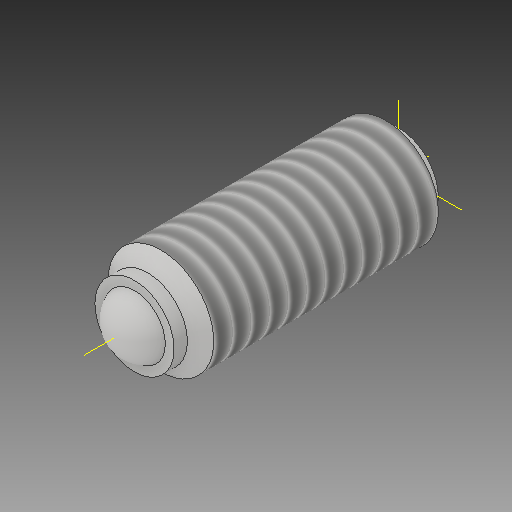
# Autodesk Inventor part: wkret_z_kulka
Saved by Autodesk Inventor 2019.4 (Build 234330000, 330)
## iProperties
Created: 2019-05-25
Part Number: wkret_z_kulka
Material: Ogólne
Document SubType Name: Modeling
Designer: Esterka
Density: 1 g/cm^3
Appearance: Domyślne
Author: Esterka
Autodesk Inventor part; units mm, degrees
ref_plane "YZ Plane" through (0, 0, 0) normal (1, 0, 0) x (0, 1, 0)
ref_plane "XZ Plane" through (0, 0, 0) normal (0, 1, 0) x (-1, 0, 0)
ref_plane "XY Plane" through (0, 0, 0) normal (0, 0, 1) x (1, 0, 0)
sketch "Sketch1" plane through (0, 0, 0) normal (0, 0, 1) x (1, 0, 0)
  circle A0 centre (0, 0) radius 2
  dimension "d0" = 4
  constraints: 1 centre point, 1 coincident
  measures "d0" diameter of A0
extrude "Extrusion1" add sketch "Sketch1" along normal blind 10
thread "Thread1" size "M4x0.7" class "6g" standard "ISO Metric profile" full length
sketch "Sketch2" plane through (0, 0, 0) normal (0, 1, 0) x (-1, 0, 0)
  line L0 (2, 0) -> (2, 10) projected
  line L1 (2, 0) -> (2, 0.5)
  line L2 (2, 0.5) -> (1.5, 0)
  line L3 (-2, 0) -> (2, 0) projected
  line L4 (2, 10) -> (-2, 10) projected
  line L5 (2, 10) -> (1.5, 10)
  line L6 (1.5, 10) -> (1.5, 9.5)
  line L7 (1.5, 9.5) -> (2, 9)
  line L8 (0, -2) -> (0, 12) projected
  point P0 (0, 0)
  dimension "d5" = 0.5
  dimension "d6" = 45
  dimension "d7" = 0.5
  dimension "d8" = 0.5
  constraints: 10 end point, 5 point on line, 1 perpendicular
  measures "d5" distance of L1.start L1.end
  measures "d6" angle of L0 L2
  measures "d7" distance of L0.end L5.end
  measures "d8" distance of L5.end L6.end
revolve "Revolution1" cut sketch "Sketch2" angle 360 about axis through (0, 0, -10) along (0, 0, 1) contours L3 L2 L0 | L7 L6 L4 L0
sketch "Sketch3" plane through (0, 0, 0) normal (0, 1, 0) x (-1, 0, 0)
  arc A0 (0, 10.8) -> (-1.1662, 10) centre (0, 9.55) ccw
  line L0 (1.5, 10) -> (-1.5, 10) projected
  line L1 (0, 10.8) -> (0, 10)
  line L2 (0, -2.1962) -> (0, 13.1769) projected
  point P0 (0, 0)
  dimension "d11" = 2.5
  constraints: 2 end point, 2 point on circle, 1 centre point, 1 midpoint, 1 point on line
  measures "d11" diameter of A0
revolve "Revolution2" add sketch "Sketch3" angle 360 about axis through (0, 0, -10) along (0, 0, 1)
sketch "Sketch5" plane through (0, 0, 0) normal (0, 0, -1) x (-1, 0, 0)
  circle A0 centre (0, 0) radius 1
  line L0 (0.5774, -1) -> (-0.5774, -1)
  line L1 (-0.5774, -1) -> (-1.1547, 0)
  line L2 (0.5774, -1) -> (1.1547, 0)
  line L3 (0.5774, 1) -> (-0.5774, 1)
  line L4 (-0.5774, 1) -> (-1.1547, 0)
  line L5 (0.5774, 1) -> (1.1547, 0)
  dimension "d16" = 2
  dimension "d23" = 120
  dimension "d24" = 120
  constraints: 12 end point, 3 tangent, 1 centre point, 1 coincident, 1 horizontal
  measures "d16" diameter of A0
  measures "d23" angle of L1 L0
  measures "d24" angle of L2 L0
extrude "Extrusion2" cut sketch "Sketch5" against normal blind 2
sketch "Sketch7" plane through (0, 0, 0) normal (1, 0, 0) x (0, 1, 0)
  line L0 (0, 0) -> (0, 2) projected
  line L1 (-1, 0) -> (-1, 2) projected
  line L2 (0, 2) -> (-1, 2)
  line L3 (-1, 2) -> (0, 2.5774)
  line L4 (0, 2.5774) -> (0, 2)
  line L5 (0, -2.16) -> (0, 12.96) projected
  dimension "d28" = 60
  constraints: 6 end point, 1 horizontal, 1 perpendicular
  measures "d28" angle of L4 L3
revolve "Revolution3" cut sketch "Sketch7" angle 360 about axis through (0, 0, -10) along (0, 0, 1)
body "Solid1"
